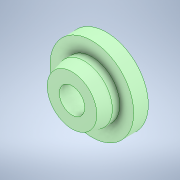
# Autodesk Inventor part: EncoderCodeWheelMount T2.5
Saved by Autodesk Inventor 2022.2 (Build 262287030, 287C)
## iProperties
Created: 2019-07-04
Part Number: EncoderCodeWheelMount T2.5
Material: Generic
Document SubType Name: Modeling
Designer: Jochen
Density: 1 g/cm^3
Appearance: Default
Sending System: SolidWorks 2017
Last Author: Felix
Last Saved: 2021-02-23
Author: Jochen
Autodesk Inventor part; units mm, degrees
ref_plane "YZ Plane" through (0, 0, 0) normal (1, 0, 0) x (0, 1, 0)
ref_plane "XZ Plane" through (0, 0, 0) normal (0, 1, 0) x (-1, 0, 0)
ref_plane "XY Plane" through (0, 0, 0) normal (0, 0, 1) x (1, 0, 0)
sketch "Sketch3" plane through (0, 0, 0) normal (0, 0, 1) x (1, 0, 0)
  line L0 (0, -6.3) -> (0, 6.3) construction
  line L1 (-6.3, 0) -> (6.3, 0) construction
  circle A0 centre (0, 0) radius 4.5
  circle A1 centre (0, 0) radius 2.05
  dimension "d42" = 9
  dimension "d45" = 4.1
  constraints: 2 centre point, 2 coincident
  measures "d42" diameter of A0
  measures "d45" diameter of A1
extrude "Extrusion5" add sketch "Sketch3" against normal blind 3.2
sketch "Sketch1" plane through (0, 0, -3.2) normal (0, 0, 1) x (1, 0, 0)
  line L0 (-10.64, 0) -> (10.64, 0) construction
  line L1 (0, -10.64) -> (0, 10.64) construction
  circle A0 centre (0, 0) radius 2.05
  circle A1 centre (0, 0) radius 3.05
  circle A2 centre (0, 0) radius 6.75
  arc A3 (0.3991, 3.7387) -> (0.581, 3.8546) centre (0.3991, 3.9394) ccw
  line L2 (0.581, 3.8546) -> (0.7391, 4.1936)
  arc A4 (1.0847, 4.3585) -> (0.7391, 4.1936) centre (1.012, 4.0663) ccw
  arc A5 (1.2398, 4.317) -> (1.0847, 4.3585) centre (0, 0) ccw
  arc A6 (1.4567, 4.0013) -> (1.2398, 4.317) centre (1.1567, 4.0275) ccw
  line L3 (1.4567, 4.0013) -> (1.4241, 3.6287)
  arc A7 (1.4241, 3.6287) -> (1.5237, 3.4373) centre (1.6241, 3.6112) ccw
  line L4 (1.5237, 3.4373) -> (2.2149, 3.0382)
  arc A8 (2.2149, 3.0382) -> (2.4305, 3.0476) centre (2.3153, 3.2121) ccw
  line L5 (2.4305, 3.0476) -> (2.7369, 3.2622)
  arc A9 (3.1187, 3.2322) -> (2.7369, 3.2622) centre (2.9096, 3.0155) ccw
  arc A10 (3.2322, 3.1187) -> (3.1187, 3.2322) centre (0, 0) ccw
  arc A11 (3.2622, 2.7369) -> (3.2322, 3.1187) centre (3.0155, 2.9096) ccw
  line L6 (3.2622, 2.7369) -> (3.0476, 2.4305)
  arc A12 (3.0476, 2.4305) -> (3.0382, 2.2149) centre (3.2121, 2.3153) ccw
  line L7 (3.0382, 2.2149) -> (3.4373, 1.5237)
  arc A13 (3.4373, 1.5237) -> (3.6287, 1.4241) centre (3.6112, 1.6241) ccw
  line L8 (3.6287, 1.4241) -> (4.0013, 1.4567)
  arc A14 (4.317, 1.2398) -> (4.0013, 1.4567) centre (4.0275, 1.1567) ccw
  arc A15 (4.3585, 1.0847) -> (4.317, 1.2398) centre (0, 0) ccw
  arc A16 (4.1936, 0.7391) -> (4.3585, 1.0847) centre (4.0663, 1.012) ccw
  line L9 (4.1936, 0.7391) -> (3.8546, 0.581)
  arc A17 (3.8546, 0.581) -> (3.7387, 0.3991) centre (3.9394, 0.3991) ccw
  line L10 (3.7387, 0.3991) -> (3.7387, -0.3991)
  arc A18 (3.7387, -0.3991) -> (3.8546, -0.581) centre (3.9394, -0.3991) ccw
  line L11 (3.8546, -0.581) -> (4.1936, -0.7391)
  arc A19 (4.3585, -1.0847) -> (4.1936, -0.7391) centre (4.0663, -1.012) ccw
  arc A20 (4.317, -1.2398) -> (4.3585, -1.0847) centre (0, 0) ccw
  arc A21 (4.0013, -1.4567) -> (4.317, -1.2398) centre (4.0275, -1.1567) ccw
  line L12 (4.0013, -1.4567) -> (3.6287, -1.4241)
  arc A22 (3.6287, -1.4241) -> (3.4373, -1.5237) centre (3.6112, -1.6241) ccw
  line L13 (3.4373, -1.5237) -> (3.0382, -2.2149)
  arc A23 (3.0382, -2.2149) -> (3.0476, -2.4305) centre (3.2121, -2.3153) ccw
  line L14 (3.0476, -2.4305) -> (3.2622, -2.7369)
  arc A24 (3.2322, -3.1187) -> (3.2622, -2.7369) centre (3.0155, -2.9096) ccw
  arc A25 (3.1187, -3.2322) -> (3.2322, -3.1187) centre (0, 0) ccw
  arc A26 (2.7416, -3.2654) -> (3.1187, -3.2322) centre (2.9096, -3.0155) ccw
  line L15 (2.7416, -3.2654) -> (2.4277, -3.0494)
  arc A27 (2.4277, -3.0494) -> (2.2142, -3.0406) centre (2.3139, -3.2148) ccw
  line L16 (2.2142, -3.0406) -> (1.5216, -3.4385)
  arc A28 (1.5216, -3.4385) -> (1.4241, -3.6287) centre (1.6241, -3.6111) ccw
  line L17 (1.4241, -3.6287) -> (1.4567, -4.0013)
  arc A29 (1.2398, -4.317) -> (1.4567, -4.0013) centre (1.1567, -4.0275) ccw
  arc A30 (1.0847, -4.3585) -> (1.2398, -4.317) centre (0, 0) ccw
  arc A31 (0.7391, -4.1936) -> (1.0847, -4.3585) centre (1.012, -4.0663) ccw
  line L18 (0.7391, -4.1936) -> (0.581, -3.8546)
  arc A32 (0.581, -3.8546) -> (0.3991, -3.7387) centre (0.3991, -3.9394) ccw
  line L19 (0.3991, -3.7387) -> (-0.3991, -3.7387)
  arc A33 (-0.3991, -3.7387) -> (-0.581, -3.8546) centre (-0.3991, -3.9394) ccw
  line L20 (-0.581, -3.8546) -> (-0.7391, -4.1936)
  arc A34 (-1.0847, -4.3585) -> (-0.7391, -4.1936) centre (-1.012, -4.0663) ccw
  arc A35 (-1.2398, -4.317) -> (-1.0847, -4.3585) centre (0, 0) ccw
  arc A36 (-1.4567, -4.0013) -> (-1.2398, -4.317) centre (-1.1567, -4.0275) ccw
  line L21 (-1.4567, -4.0013) -> (-1.4241, -3.6287)
  arc A37 (-1.4241, -3.6287) -> (-1.5237, -3.4373) centre (-1.6241, -3.6112) ccw
  line L22 (-1.5237, -3.4373) -> (-2.2149, -3.0382)
  arc A38 (-2.2149, -3.0382) -> (-2.4305, -3.0476) centre (-2.3153, -3.2121) ccw
  line L23 (-2.4305, -3.0476) -> (-2.7369, -3.2622)
  arc A39 (-3.1187, -3.2322) -> (-2.7369, -3.2622) centre (-2.9096, -3.0155) ccw
  arc A40 (-3.2322, -3.1187) -> (-3.1187, -3.2322) centre (0, 0) ccw
  arc A41 (-3.2622, -2.7369) -> (-3.2322, -3.1187) centre (-3.0155, -2.9096) ccw
  line L24 (-3.2622, -2.7369) -> (-3.0476, -2.4305)
  arc A42 (-3.0476, -2.4305) -> (-3.0382, -2.2149) centre (-3.2121, -2.3153) ccw
  line L25 (-3.0382, -2.2149) -> (-3.4373, -1.5237)
  arc A43 (-3.4373, -1.5237) -> (-3.6287, -1.4241) centre (-3.6112, -1.6241) ccw
  line L26 (-3.6287, -1.4241) -> (-4.0013, -1.4567)
  arc A44 (-4.317, -1.2398) -> (-4.0013, -1.4567) centre (-4.0275, -1.1567) ccw
  arc A45 (-4.3585, -1.0847) -> (-4.317, -1.2398) centre (0, 0) ccw
  arc A46 (-4.193, -0.7388) -> (-4.3585, -1.0847) centre (-4.0663, -1.012) ccw
  line L27 (-4.193, -0.7388) -> (-3.8544, -0.5784)
  arc A47 (-3.8544, -0.5784) -> (-3.7398, -0.4) centre (-3.9405, -0.397) ccw
  line L28 (-3.7398, -0.4) -> (-3.7386, 0.4009)
  arc A48 (-3.7386, 0.4009) -> (-3.8546, 0.581) centre (-3.9394, 0.3991) ccw
  line L29 (-3.8546, 0.581) -> (-4.1936, 0.7391)
  arc A49 (-4.3585, 1.0847) -> (-4.1936, 0.7391) centre (-4.0663, 1.012) ccw
  arc A50 (-4.317, 1.2398) -> (-4.3585, 1.0847) centre (0, 0) ccw
  arc A51 (-4.0013, 1.4567) -> (-4.317, 1.2398) centre (-4.0275, 1.1567) ccw
  line L30 (-4.0013, 1.4567) -> (-3.6287, 1.4241)
  arc A52 (-3.6287, 1.4241) -> (-3.4373, 1.5237) centre (-3.6112, 1.6241) ccw
  line L31 (-3.4373, 1.5237) -> (-3.0488, 2.1966)
  arc A53 (-3.0488, 2.1966) -> (-3.0462, 2.4327) centre (-3.2098, 2.3164) ccw
  line L32 (-3.0462, 2.4327) -> (-3.2595, 2.733)
  arc A54 (-3.2322, 3.1187) -> (-3.2595, 2.733) centre (-3.0155, 2.9096) ccw
  arc A55 (-3.1187, 3.2322) -> (-3.2322, 3.1187) centre (0, 0) ccw
  arc A56 (-2.7369, 3.2622) -> (-3.1187, 3.2322) centre (-2.9096, 3.0155) ccw
  line L33 (-2.7369, 3.2622) -> (-2.4305, 3.0476)
  arc A57 (-2.4305, 3.0476) -> (-2.2149, 3.0382) centre (-2.3153, 3.2121) ccw
  line L34 (-2.2149, 3.0382) -> (-1.5237, 3.4373)
  arc A58 (-1.5237, 3.4373) -> (-1.4241, 3.6287) centre (-1.6241, 3.6112) ccw
  line L35 (-1.4241, 3.6287) -> (-1.4567, 4.0013)
  arc A59 (-1.2398, 4.317) -> (-1.4567, 4.0013) centre (-1.1567, 4.0275) ccw
  arc A60 (-1.0847, 4.3585) -> (-1.2398, 4.317) centre (0, 0) ccw
  arc A61 (-0.7391, 4.1936) -> (-1.0847, 4.3585) centre (-1.012, 4.0663) ccw
  line L36 (-0.7391, 4.1936) -> (-0.581, 3.8546)
  arc A62 (-0.581, 3.8546) -> (-0.3991, 3.7387) centre (-0.3991, 3.9394) ccw
  line L37 (-0.3991, 3.7387) -> (0.3991, 3.7387)
  circle A63 centre (0, 0) radius 7.6
  circle A64 centre (0, 0) radius 4.4915 construction
  arc A65 (0.3991, 3.9137) -> (0.4224, 3.9285) centre (0.3991, 3.9394) ccw
  arc A66 (1.5984, 3.6134) -> (1.6112, 3.5889) centre (1.6241, 3.6112) ccw
  arc A67 (2.3024, 3.1898) -> (2.3301, 3.191) centre (2.3153, 3.2121) ccw
  arc A68 (3.191, 2.3301) -> (3.1898, 2.3024) centre (3.2121, 2.3153) ccw
  arc A69 (3.5889, 1.6112) -> (3.6134, 1.5984) centre (3.6112, 1.6241) ccw
  arc A70 (3.9285, 0.4224) -> (3.9137, 0.3991) centre (3.9394, 0.3991) ccw
  arc A71 (3.9137, -0.3991) -> (3.9285, -0.4224) centre (3.9394, -0.3991) ccw
  arc A72 (3.6134, -1.5984) -> (3.5889, -1.6112) centre (3.6112, -1.6241) ccw
  arc A73 (3.1898, -2.3024) -> (3.191, -2.3301) centre (3.2121, -2.3153) ccw
  arc A74 (-2.3024, -3.1898) -> (-2.3301, -3.191) centre (-2.3153, -3.2121) ccw
  arc A75 (-3.191, -2.3301) -> (-3.1898, -2.3024) centre (-3.2121, -2.3153) ccw
  arc A76 (-3.5889, -1.6112) -> (-3.6134, -1.5984) centre (-3.6112, -1.6241) ccw
  arc A77 (-3.9295, -0.4203) -> (-3.9148, -0.3958) centre (-3.9405, -0.397) ccw
  arc A78 (-3.9136, 0.3991) -> (-3.9285, 0.4224) centre (-3.9394, 0.3991) ccw
  arc A79 (-3.6134, 1.5984) -> (-3.5889, 1.6112) centre (-3.6112, 1.6241) ccw
  arc A80 (-3.1846, 2.3113) -> (-3.1888, 2.3313) centre (-3.2098, 2.3164) ccw
  arc A81 (-2.3301, 3.191) -> (-2.3024, 3.1898) centre (-2.3153, 3.2121) ccw
  arc A82 (-1.6112, 3.5889) -> (-1.5984, 3.6134) centre (-1.6241, 3.6112) ccw
  arc A83 (-0.4224, 3.9285) -> (-0.3991, 3.9137) centre (-0.3991, 3.9394) ccw
  line L38 (-2.3128, -3.2704) -> (-1.6759, -3.6381)
  line L39 (-1.6759, -3.6381) -> (-1.7058, -3.9795)
  arc A84 (-1.7058, -3.9795) -> (-1.3089, -4.5572) centre (-1.1567, -4.0275) ccw
  arc A85 (-1.3089, -4.5572) -> (-1.1451, -4.6011) centre (0, 0) ccw
  arc A86 (-1.1451, -4.6011) -> (-0.5125, -4.2992) centre (-1.012, -4.0663) ccw
  line L40 (-0.5125, -4.2992) -> (-0.3677, -3.9887)
  line L41 (-0.3677, -3.9887) -> (0.3677, -3.9887)
  line L42 (0.3677, -3.9887) -> (0.5125, -4.2992)
  arc A87 (0.5125, -4.2992) -> (1.1451, -4.6011) centre (1.012, -4.0663) ccw
  arc A88 (1.1451, -4.6011) -> (1.3089, -4.5572) centre (0, 0) ccw
  arc A89 (1.3089, -4.5572) -> (1.7058, -3.9795) centre (1.1567, -4.0275) ccw
  line L43 (1.7058, -3.9795) -> (1.6759, -3.6381)
  line L44 (1.6759, -3.6381) -> (2.3116, -3.273)
  line L45 (2.3116, -3.273) -> (2.5935, -3.467)
  arc A90 (2.5935, -3.467) -> (3.2923, -3.4121) centre (2.9096, -3.0155) ccw
  arc A91 (3.2923, -3.4121) -> (3.4121, -3.2923) centre (0, 0) ccw
  arc A92 (3.4121, -3.2923) -> (3.467, -2.5935) centre (3.0155, -2.9096) ccw
  line L46 (3.467, -2.5935) -> (3.2704, -2.3128)
  line L47 (3.2704, -2.3128) -> (3.6381, -1.6759)
  line L48 (3.6381, -1.6759) -> (3.9795, -1.7058)
  arc A93 (3.9795, -1.7058) -> (4.5572, -1.3089) centre (4.0275, -1.1567) ccw
  arc A94 (4.5572, -1.3089) -> (4.6011, -1.1451) centre (0, 0) ccw
  arc A95 (4.6011, -1.1451) -> (4.2992, -0.5125) centre (4.0663, -1.012) ccw
  line L49 (4.2992, -0.5125) -> (3.9887, -0.3677)
  line L50 (3.9887, -0.3677) -> (3.9887, 0.3677)
  line L51 (3.9887, 0.3677) -> (4.2992, 0.5125)
  arc A96 (4.2992, 0.5125) -> (4.6011, 1.1451) centre (4.0663, 1.012) ccw
  arc A97 (4.6011, 1.1451) -> (4.5572, 1.3089) centre (0, 0) ccw
  arc A98 (4.5572, 1.3089) -> (3.9795, 1.7058) centre (4.0275, 1.1567) ccw
  line L52 (3.9795, 1.7058) -> (3.6381, 1.6759)
  line L53 (3.6381, 1.6759) -> (3.2704, 2.3128)
  line L54 (3.2704, 2.3128) -> (3.467, 2.5935)
  arc A99 (3.467, 2.5935) -> (3.4121, 3.2923) centre (3.0155, 2.9096) ccw
  arc A100 (3.4121, 3.2923) -> (3.2923, 3.4121) centre (0, 0) ccw
  arc A101 (3.2923, 3.4121) -> (2.5935, 3.467) centre (2.9096, 3.0155) ccw
  line L55 (2.5935, 3.467) -> (2.3128, 3.2704)
  line L56 (2.3128, 3.2704) -> (1.6759, 3.6381)
  line L57 (1.6759, 3.6381) -> (1.7058, 3.9795)
  arc A102 (1.7058, 3.9795) -> (1.3089, 4.5572) centre (1.1567, 4.0275) ccw
  arc A103 (1.3089, 4.5572) -> (1.1451, 4.6011) centre (0, 0) ccw
  arc A104 (1.1451, 4.6011) -> (0.5125, 4.2992) centre (1.012, 4.0663) ccw
  line L58 (0.5125, 4.2992) -> (0.3677, 3.9887)
  line L59 (0.3677, 3.9887) -> (-0.3677, 3.9887)
  line L60 (-0.3677, 3.9887) -> (-0.5125, 4.2992)
  arc A105 (-0.5125, 4.2992) -> (-1.1451, 4.6011) centre (-1.012, 4.0663) ccw
  arc A106 (-1.1451, 4.6011) -> (-1.3089, 4.5572) centre (0, 0) ccw
  arc A107 (-1.3089, 4.5572) -> (-1.7058, 3.9795) centre (-1.1567, 4.0275) ccw
  line L61 (-1.7058, 3.9795) -> (-1.6759, 3.6381)
  line L62 (-1.6759, 3.6381) -> (-2.3128, 3.2704)
  line L63 (-2.3128, 3.2704) -> (-2.5935, 3.467)
  arc A108 (-2.5935, 3.467) -> (-3.2923, 3.4121) centre (-2.9096, 3.0155) ccw
  arc A109 (-3.2923, 3.4121) -> (-3.4121, 3.2923) centre (0, 0) ccw
  arc A110 (-3.4121, 3.2923) -> (-3.467, 2.5935) centre (-3.0155, 2.9096) ccw
  line L64 (-3.467, 2.5935) -> (-3.2691, 2.3149)
  line L65 (-3.2691, 2.3149) -> (-3.6381, 1.6759)
  line L66 (-3.6381, 1.6759) -> (-3.9795, 1.7058)
  arc A111 (-3.9795, 1.7058) -> (-4.5572, 1.3089) centre (-4.0275, 1.1567) ccw
  arc A112 (-4.5572, 1.3089) -> (-4.6011, 1.1451) centre (0, 0) ccw
  arc A113 (-4.6011, 1.1451) -> (-4.2992, 0.5125) centre (-4.0663, 1.012) ccw
  line L67 (-4.2992, 0.5125) -> (-3.9887, 0.3677)
  line L68 (-3.9887, 0.3677) -> (-3.9897, -0.3658)
  line L69 (-3.9897, -0.3658) -> (-4.2992, -0.5125)
  arc A114 (-4.2992, -0.5125) -> (-4.6011, -1.1451) centre (-4.0663, -1.012) ccw
  arc A115 (-4.6011, -1.1451) -> (-4.5572, -1.3089) centre (0, 0) ccw
  arc A116 (-4.5572, -1.3089) -> (-3.9795, -1.7058) centre (-4.0275, -1.1567) ccw
  line L70 (-3.9795, -1.7058) -> (-3.6381, -1.6759)
  line L71 (-3.6381, -1.6759) -> (-3.2704, -2.3128)
  line L72 (-3.2704, -2.3128) -> (-3.467, -2.5935)
  arc A117 (-3.467, -2.5935) -> (-3.4121, -3.2923) centre (-3.0155, -2.9096) ccw
  arc A118 (-3.4121, -3.2923) -> (-3.2923, -3.4121) centre (0, 0) ccw
  arc A119 (-3.2923, -3.4121) -> (-2.5935, -3.467) centre (-2.9096, -3.0155) ccw
  line L73 (-2.5935, -3.467) -> (-2.3128, -3.2704)
  circle A120 centre (0, 0) radius 2.05 construction
  dimension "d5" = 13.5
  dimension "d40" = 0.25
  dimension "d41" = 6.1
  dimension "d49" = 0.85
  constraints: 230 point on circle, 144 end point, 119 centre point, 3 coincident, 2 concentric, 74 other
  measures "d5" diameter of A2
  measures "d40" distance between parallel lines of L22 L38
  measures "d41" diameter of A1
  measures "d49" radial gap between concentric circles of A63 A2
extrude "Extrusion2" add sketch "Sketch1" against normal blind 1.2 from surface at 0 contours A1 | A2 | A3 L2 A4 A5 A6 L3 A7 L4 A8 L5 A9 A10 A11 L6 A12 L7 A13 L8 A14 A15 A16 L9 A17 L10 A18 L11 A19 A20 A21 L12 A22 L13 A23 L14 A24 A25 A26 L15 A27 L16 A28 L17 A29 A30 A31 L18 A32 L19 A33 L20 A34 A35 A36 L21 A37 L22 A38 L23 A39 A40 A41 L24 A42 L25 A43 L26 A44 A45 A46 L27 A47 L28 A48 L29 A49 A50 A51 L30 A52 L31 A53 L32 A54 A55 A56 L33 A57 L34 A58 L35 A59 A60 A61 L36 A62 L37 | L73 A119 A118 A117 L72 L71 L70 A116 A115 A114 L69 L68 L67 A113 A112 A111 L66 L65 L64 A110 A109 A108 L63 L62 L61 A107 A106 A105 L60 L59 L58 A104 A103 A102 L57 L56 L55 A101 A100 A99 L54 L53 L52 A98 A97 A96 L51 L50 L49 A95 A94 A93 L48 L47 L46 A92 A91 A90 L45 L44 L43 A89 A88 A87 L42 L41 L40 A86 A85 A84 L39 L38
extrude "Extrusion4" add sketch "Sketch1" against normal blind 1.4 from surface at -1.2 contours A2
chamfer "Chamfer1" distance 0.5 distance2 0.25 1 edges at (-6.75, 0, -5.8) measured on face at (-6.25, 0, -5.8)
chamfer "Chamfer2" distance 0.2 distance2 0.8 1 edges at (-2.05, 0, -4.4) measured on face at (-2.55, 0, -4.4)
chamfer "Chamfer5" distance 0.5 distance2 2 1 edges at (-4.5, 0, 0) measured on face at (-4, 0, 0)
body "Solid1"
body "Solid5"
